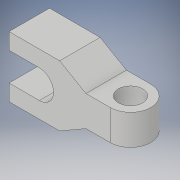
# Autodesk Inventor part: 複習一
Saved by Autodesk Inventor 2017 (Build 210142000, 142)
## iProperties
Part Number: 複習一
Material: 一般
Document SubType Name: Modeling
Designer: user
Density: 1 g/cm^3
Appearance: 預設
Author: user
Autodesk Inventor part; units mm, degrees
ref_plane "YZ Plane" through (0, 0, 0) normal (1, 0, 0) x (0, 1, 0)
ref_plane "XZ Plane" through (0, 0, 0) normal (0, 1, 0) x (-1, 0, 0)
ref_plane "XY Plane" through (0, 0, 0) normal (0, 0, 1) x (1, 0, 0)
sketch "草圖1" plane through (0, 0, 0) normal (0, 0, 1) x (1, 0, 0)
  line L0 (0, 0) -> (0, 16)
  line L1 (0, 16) -> (30, 16)
  line L2 (30, 44) -> (0, 44)
  line L3 (0, 44) -> (0, 60)
  line L4 (0, 60) -> (50, 60)
  line L5 (50, 60) -> (75.9808, 45)
  line L6 (75.9808, 45) -> (120, 45)
  line L7 (120, 45) -> (120, 15)
  line L8 (120, 15) -> (75.9808, 15)
  line L9 (75.9808, 15) -> (50, 0)
  line L10 (50, 0) -> (0, 0)
  arc A0 (30, 16) -> (30, 44) centre (30, 30) ccw
  dimension "d0" = 60
  dimension "d1" = 50
  dimension "d3" = 30
  dimension "d5" = 30
  dimension "d6" = 120
  dimension "d8" = 28
  dimension "d10" = 16
  dimension "d13" = 50
  dimension "d25" = 45
  dimension "d26" = 30
  dimension "d27" = 30
  constraints: 22 end point, 5 perpendicular, 3 parallel, 2 point on circle, 2 tangent, 1 centre point, 1 collinear, 1 horizontal, 1 vertical, 1 vertical alignment
  measures "d0" distance between parallel lines of L10 L4
  measures "d1" distance of L3.end L4.end
  measures "d3" angle of L5 L4
  measures "d5" angle of L10 L9
  measures "d6" distance between parallel lines of L7 L0
  measures "d8" distance between parallel lines of L2 L1
  measures "d10" distance between parallel lines of L10 L1
  measures "d13" distance of L9.end L0.start
  measures "d25" distance between parallel lines of L10 L6
  measures "d26" distance between parallel lines of L8 L6
  measures "d27" distance from line of L3 A0.centre
extrude "擠出1" add sketch "草圖1" along normal blind 40
fillet "圓角1" radius 20 2 edges at (120, 30, 40) (120, 30, 0)
sketch "草圖2" plane through (75.9808, 45, 40) normal (0, 1, 0) x (1, 0, 0)
  arc A0 (24.0192, 0) -> (24.0192, 40) centre (24.0192, 20) ccw projected
  circle A1 centre (24.0192, 20) radius 12
  point P0 (-75.9808, 40)
  dimension "d49" = 24
  constraints: 1 centre point, 1 coincident
  measures "d49" diameter of A1
extrude "擠出2" cut sketch "草圖2" against normal blind 40
